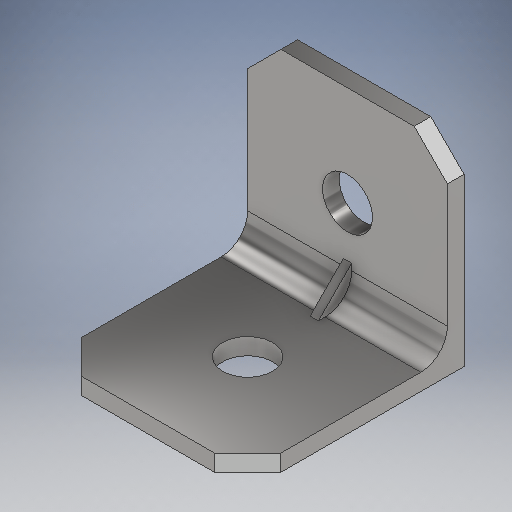
# Autodesk Inventor part: PARAMETRIC L-BRAKET
Saved by Autodesk Inventor 2025.2 (Build 292293000, 293)
## iProperties
Created: 2025-02-12
Part Number: PARAMETRIC L-BRAKET
Material: Generic
Document SubType Name: Modeling
Designer: Anna
Density: 1 g/cm^3
Appearance: Default
RuleStatus: InUse
Author: Anna
Autodesk Inventor part; units mm, degrees
ref_plane "YZ Plane" through (0, 0, 0) normal (1, 0, 0) x (0, 1, 0)
ref_plane "XZ Plane" through (0, 0, 0) normal (0, 1, 0) x (-1, 0, 0)
sketch "Sketch1" plane through (0, 0, 0) normal (0, 1, 0) x (-1, 0, 0)
  line L0 (57.15, 0) -> (-19.05, 0)
  line L1 (-19.05, 0) -> (-19.05, -76.2)
  line L2 (-19.05, -76.2) -> (57.15, -76.2)
  line L3 (57.15, -76.2) -> (57.15, 0)
  point P0 (0, 0)
  dimension "d0" = 76.2
  dimension "d1" = 76.2
  constraints: 8 end point, 2 parallel, 1 horizontal, 1 perpendicular
  measures "d0" distance of L2.end L0.start
  measures "d1" distance of L1.end L2.end
extrude "BOTTOM" add sketch "Sketch1" along normal blind 6.35
sketch "Sketch2" plane through (19.05, 0, -76.2) normal (0, 0, -1) x (-1, 0, 0)
  line L0 (0, 0) -> (76.2, 0)
  line L1 (76.2, 0) -> (76.2, 76.2)
  line L2 (76.2, 76.2) -> (0, 76.2)
  line L3 (0, 76.2) -> (0, 0)
  point P0 (19.05, 0)
  dimension "d4" = 76.2
  dimension "d5" = 76.2
  constraints: 8 end point, 2 parallel, 1 horizontal, 1 perpendicular
  measures "d4" distance of L1.end L2.end
  measures "d5" distance of L0.end L1.end
extrude "SIDE" add sketch "Sketch2" along normal blind 6.35
sketch "Sketch3" plane through (0, 6.35, 0) normal (0, 1, 0) x (1, 0, 0)
  circle A0 centre (-19.05, 38.1) radius 9.525
  line L0 (-57.15, 76.2) -> (19.05, 76.2) projected
  line L1 (-57.15, 76.2) -> (-57.15, 0) projected
  point P0 (0, 0)
  point P1 (-44.45, 76.2)
  point P2 (6.35, 76.2)
  point P3 (-57.15, 12.7)
  dimension "d9" = 19.05
  dimension "d10" = 38.1
  dimension "d11" = 38.1
  constraints: 1 centre point
  measures "d9" diameter of A0
  measures "d10" distance from line of L0 A0.centre
  measures "d11" distance from line of L1 A0.centre
extrude "HOLE BOTT" cut sketch "Sketch3" against normal blind 6.35
sketch "Sketch4" plane through (19.05, 0, -76.2) normal (0, 0, 1) x (1, 0, 0)
  circle A0 centre (-38.1, 38.1) radius 9.525
  line L0 (-76.2, 76.2) -> (0, 76.2) projected
  line L1 (0, 76.2) -> (0, 6.35) projected
  point P0 (-19.05, 0)
  point P1 (-63.5, 76.2)
  point P2 (-12.7, 76.2)
  point P3 (0, 63.5)
  dimension "d14" = 19.05
  dimension "d15" = 38.1
  dimension "d16" = 38.1
  constraints: 1 centre point
  measures "d14" diameter of A0
  measures "d15" distance from line of L0 A0.centre
  measures "d16" distance from line of L1 A0.centre
extrude "HOLE SIDE" cut sketch "Sketch4" against normal blind 6.35
chamfer "CHM TOP" distance 12.7 angle 45 2 edges at (19.05, 76.2, -79.375) (-57.15, 76.2, -79.375)
ref_plane "Work Plane1" through (-19.05, 6.35, -76.2) normal (-1, 0, 0) x (0, 0, 1)
sketch "Sketch6" plane through (-19.05, 6.35, -76.2) normal (-1, 0, 0) x (0, 0, 1)
  line L0 (0, 0) -> (12.7, 0)
  line L1 (12.7, 0) -> (0, 12.7)
  line L2 (0, 12.7) -> (0, 0)
  point P0 (76.2, -6.35)
  dimension "d25" = 12.7
  dimension "d27" = 12.7
  constraints: 6 end point, 1 vertical
  measures "d25" distance of L0.start L0.end
  measures "d27" distance of L1.end L0.start
extrude "BRACE" add sketch "Sketch6" along normal mid plane 3.175
fillet "Fillet1" radius 10.16 2 edges at (-38.8937, 6.35, -76.2) (0.7938, 6.35, -76.2)
chamfer "CHM BOTT" distance 12.7 angle 45 2 edges at (-57.15, 3.175, 0) (19.05, 3.175, 0)
equation "\"d0\" = L"
equation "\"d1\" = w"
equation "\"d2\" = HT"
equation "\"d4\" = w"
equation "\"d5\" = L"
equation "\"d6\" = HT"
equation "\"d9\" = HL"
equation "\"d10\" = 0.5 * L"
equation "\"d11\" = 0.5 * w"
equation "\"d12\" = HT"
equation "\"d14\" = HL"
equation "\"d15\" = 0.5 * L"
equation "\"d16\" = 0.5 * w"
equation "\"d17\" = HT"
equation "\"d19\" = CHM"
equation "\"d28\" = 0.5 * HT"
equation "\"d31\" = CHM"
equation "\"d30\" = FL"
equation "\"L\" = 76.2"
equation "\"w\" = 76.2"
equation "\"HT\" = 6.35"
equation "\"CHM\" = 12.7"
equation "\"HL\" = 19.05"
equation "\"d24\" = -0.5 * w"
equation "\"FL\" = 10.16"
body "Solid1"
